Autodesk Fusion 360 part; units mm, degrees
(part 2 of 2)
component "case back panel" placed x (1, 0, 0) y (0, 1, 0) z (0, 0, 1) at (0, 0, 0)
component "case foot" placed x (1, 0, 0) y (0, 1, 0) z (0, 0, 1) at (0, 0, 0)
equation "BORDER_W = 18.5 mm"
equation "SHELL = 1.8 mm"
equation "d105 = BORDER_W"
equation "d106 = BORDER_W"
equation "d108 = BORDER_H"
equation "d109 = -SHELL"
equation "d110 = -( ( SHELL / 2 ) + TOLERANCE )"
equation "TOLERANCE = 0.1 mm"
equation "d116 = -2 * TOLERANCE"
equation "d117 = -2 * TOLERANCE"
equation "d118 = -2 * TOLERANCE"
equation "d119 = -2 * TOLERANCE"
equation "CHAMFER = 0.6 mm"
equation "d127 = -( SHELL / 2 ) + TOLERANCE"
equation "d128 = TOLERANCE"
equation "DEPTH = 15 mm"
equation "d136 = TOLERANCE"
equation "d138 = -SHELL"
equation "d147 = CHAMFER"
equation "CATCH_WIDTH = 75 mm"
equation "d155 = CATCH_WIDTH + 1 mm"
equation "d158 = TOLERANCE / 2"
equation "LEG_WIDTH = 10 mm"
equation "d216 = SHELL"
equation "d218 = SHELL"
equation "d225 = SHELL - 2 * TOLERANCE"
equation "d226 = TOLERANCE"
equation "d228 = CHAMFER"
equation "d229 = 2 * TOLERANCE"
equation "d230 = 1.2 mm + 2 * TOLERANCE"
equation "d239 = 2 * TOLERANCE"
named bodies: "case_front", "case_rear", "case_foot", "case_back_panel"
